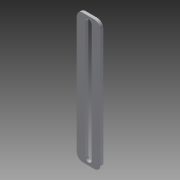
# Autodesk Inventor part: back brace mount
Saved by Autodesk Inventor 2013 (Build 170138000, 138)
## iProperties
Created: 2013-02-04
Part Number: back brace mount
Material: Aluminum 6061
Document SubType Name: Sheet Metal
Designer: Arpan
Density: 1 g/cm^3
Sheet Metal Rule: Default
Mass: 4.46226 g
Surface Area: 36.0407 cm^2
Volume: 4.46226 cm^3
Author: Arpan
Autodesk Inventor part; units mm, degrees
ref_plane "YZ Plane" through (0, 0, 0) normal (1, 0, 0) x (0, 1, 0)
ref_plane "XZ Plane" through (0, 0, 0) normal (0, 1, 0) x (-1, 0, 0)
ref_plane "XY Plane" through (0, 0, 0) normal (0, 0, 1) x (1, 0, 0)
sketch "Sketch1" plane through (0, 0, 0) normal (0, 0, 1) x (1, 0, 0)
  line L0 (36.9289, 8.8897) -> (11.5289, 8.8897)
  line L1 (36.9289, 148.5897) -> (36.9289, 8.8897)
  line L2 (11.5289, 148.5897) -> (36.9289, 148.5897)
  line L3 (20.8517, 15.2397) -> (20.8517, 142.2397)
  arc A0 (27.6081, 142.2397) -> (20.8517, 142.2397) centre (24.2299, 142.2397) ccw
  line L4 (27.6081, 142.2397) -> (27.6081, 15.2397)
  arc A1 (20.8517, 15.2397) -> (27.6081, 15.2397) centre (24.2299, 15.2397) ccw
  line L5 (36.9289, 148.5897) -> (11.5289, 148.5897)
  line L6 (11.5289, 148.5897) -> (11.5289, 8.8897)
  point P0 (0, 0)
  point P1 (0, 0)
  dimension "d0" = 25.4
  dimension "d2" = 139.7
  dimension "d5" = 6.35
  dimension "d6" = 6.35
  dimension "d7" = 3.3782
  dimension "d8" = 6.7564
  dimension "d9" = 3.3782
  measures "d0" distance of L5.end L5.start
  measures "d2" distance of L5.end L6.end
  measures "d6" distance from line of L5 A0.centre
  measures "d7" radius of A0
  measures "d8" distance between parallel lines of L4 L3
  measures "d9" radius of A1
extrude "Plate1" add sketch "Sketch1" along normal blind 3.175
fillet "Corner Round1" radius 6.35 4 edges at (36.9289, 148.5897, 1.5875) (11.5289, 148.5897, 1.5875) (36.9289, 8.8897, 1.5875) (11.5289, 8.8897, 1.5875)
equation "\"BendRadius\" = Thickness"
equation "\"BendReliefWidth\" = Thickness"
equation "\"BendReliefDepth\" = 0.5 * Thickness"
equation "\"CornerReliefSize\" = 4 * Thickness"
equation "\"MinimumRemnant\" = 2 * Thickness"
equation "\"TransitionRadius\" = BendRadius"
equation "\"JacobiRadiusSize\" = BendRadius"
equation "\"GapSize\" = Thickness"
equation "\"d1\" = BendRadius"
equation "\"Thickness\" = 3.175"
body "Solid1"
